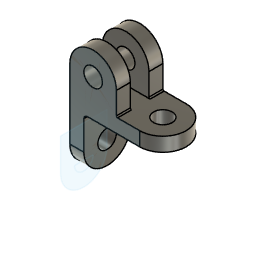
ORTHOGRAPHIC PROJECTIONS_MODEL_2 (Autodesk Fusion 360 design; units mm, degrees)
Autodesk Fusion 360 part; units mm, degrees
sketch "Sketch1" plane through (0, 0, 0) normal (0, 1, 0) x (1, 0, 0)
  circle A0 centre (0, -20) radius 8
  arc A1 (-20, -20) -> (20, -20) centre (0, -20) ccw
  line L0 (20, -20) -> (20, 0)
  line L1 (40, 12) -> (20, 12)
  line L2 (20, 12) -> (-8, 12)
  line L3 (-20, -20) -> (-20, 40)
  line L4 (-8, 12) -> (-8, 40)
  line L5 (-8, 40) -> (-20, 40)
  line L6 (40, 0) -> (40, 12)
  line L7 (20, 0) -> (40, 0)
  dimension "d1" = 20
  dimension "d2" = 16
  dimension "d3" = 20
  dimension "d7" = 28
  dimension "d8" = 60
  constraint coincident A0.centre A1.centre
  constraint tangent A1 L0
  constraint vertical L0
  constraint parallel L1 L2
  constraint perpendicular L2 L3
  constraint perpendicular L2 L4
  constraint perpendicular L3 L5
  constraint perpendicular L6 L7
  measures "d1" distance of origin A0.centre
  measures "d2" diameter of A0
  measures "d3" radius of A1
  measures "d7" distance of L1.end L2.end
  measures "d8" distance of A1.start L3.end
extrude "Extrude1" add sketch "Sketch1" against normal blind 40
sketch "Sketch2" plane through (0, 0, 0) normal (0, 0, 1) x (-1, 0, 0)
  line L0 (-40, 0) -> (-20, 0)
  line L1 (-20, 0) -> (-20, 40)
  line L2 (-20, 40) -> (-40, 40)
  line L3 (-40, 40) -> (-40, 0)
  arc A0 (-40, 40) -> (-40, 0) centre (-40, 20) ccw
  constraint tangent L2 A0
extrude "Extrude2" add sketch "Sketch2" against normal blind 12 contours L3 A0
sketch "Sketch3" plane through (-8, 0, 0) normal (1, 0, 0) x (0, 1, 0)
  line L0 (0, -40) -> (0, -12)
  line L1 (0, -12) -> (-40, -12)
  line L2 (-40, -12) -> (-40, -40)
  line L3 (-40, -40) -> (0, -40)
  arc A0 (-40, -40) -> (0, -40) centre (-20, -40) ccw
  circle A1 centre (-20, -40) radius 8
  dimension "d15" = 16
  constraint tangent L0 A0
  constraint tangent L2 A0
  constraint coincident L0.start L3.end
  constraint concentric A0 A1
  measures "d15" diameter of A1
extrude "Extrude3" add sketch "Sketch3" against normal blind 12 contours L3 A0 A1
sketch "Sketch4" plane through (-8, 0, 0) normal (1, 0, 0) x (0, 1, 0)
  line L0 (0, -40) -> (0, -12)
  line L1 (0, -12) -> (-40, -12)
  line L2 (-40, -12) -> (-40, -40)
  arc A0 (-40, -40) -> (0, -40) centre (-20, -40) ccw
  arc A1 (-28, -40) -> (-12, -40) centre (-20, -40) ccw
  line L3 (-28, -40) -> (-12, -40)
hole "Hole1" at (-8, -20, -40) direction (-1, 0, 0) diameter 16 depth 12 tip angle 118
sketch "Sketch5" plane through (0, 0, 0) normal (0, 0, 1) x (-1, 0, 0)
  line L0 (-40, 0) -> (-20, 0)
  line L1 (-20, 0) -> (-20, 40)
  line L2 (-20, 40) -> (-40, 40)
  arc A0 (-40, 40) -> (-40, 0) centre (-40, 20) ccw
  circle A1 centre (-40, 20) radius 8
  dimension "d21" = 16
  constraint concentric A0 A1
  measures "d21" diameter of A1
extrude "Extrude4" cut sketch "Sketch5" against normal blind 12 contours A1
sketch "Sketch6" plane through (-20, 0, 0) normal (-1, 0, 0) x (0, -1, 0)
  circle A0 centre (20, -40) radius 8
  arc A1 (0, -40) -> (40, -40) centre (20, -40) ccw
  line L0 (40, -40) -> (40, 20)
  line L1 (40, 20) -> (0, 20)
  line L2 (0, 20) -> (0, -40)
  line L3 (0, 0) -> (12, 0)
  line L4 (12, 0) -> (28, 0)
  line L5 (28, 0) -> (28, 43.8644)
  line L6 (28, 43.8644) -> (12, 43.8644)
  line L7 (12, 43.8644) -> (12, 0)
  dimension "d24" = 12
  dimension "d25" = 16
  constraint coincident L3.start origin
  constraint perpendicular L2 L3
  constraint horizontal L4
  constraint vertical L5
  constraint horizontal L6
  constraint vertical L7
  measures "d24" distance of L3.start L3.end
  measures "d25" distance of L3.end L4.end
extrude "Extrude5" cut sketch "Sketch6" against normal blind 40 contours L1 L4 L5 L7 | L1 L5 L6 L7
fillet "Fillet1" radius 3 1 edges at (-8, -20, -12)
fillet "Fillet2" radius 1 1 edges at (20, -34, 0)
fillet "Fillet3" radius 1 1 edges at (20, -6, 0)
move_body "Move1" bodies 1 to x (1, 0, 0) y (0, 1, 0) z (0, 0, 1) at (0, 20, 0)
move_body "Move2" bodies 1 to x (1, 0, 0) y (0, 1, 0) z (0, 0, 1) at (0, 0, 6)
sketch "Sketch7" plane through (0, -20, 0) normal (0, -1, 0) x (1, 0, 0)
  circle A0 centre (0, 26) radius 8
  arc A1 (20, 26) -> (-20, 26) centre (0, 26) ccw
  line L0 (-20, 26) -> (-20, -34)
  line L1 (-20, -34) -> (-8, -34)
  line L2 (-8, -34) -> (-8, -9)
  arc A2 (-5, -6) -> (-8, -9) centre (-5, -9) ccw
  line L3 (-5, -6) -> (40, -6)
  line L4 (40, -6) -> (40, 6)
  line L5 (40, 6) -> (21, 6)
  arc A3 (20, 7) -> (21, 6) centre (21, 7) ccw
  line L6 (20, 7) -> (20, 26)
